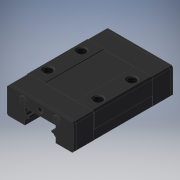
# Autodesk Inventor part: C-MLGB9
Saved by Autodesk Inventor 2019 (Build 230136000, 136)
## iProperties
Created: 2023-11-06
Part Number: C-MLGB9
Material: Generic
Catalog Web Link: www.cadenas.de
Description: C-MLGB, E-GMLGB-Economy Miniature Liner guide - Standard type - Single Block Product
Vendor: MISUMI
Document SubType Name: Modeling
Designer: psAdmin
Manufacturer: MISUMI
Mass: 3.14177 g
Surface Area: 23.9367 cm^2
Volume: 3.14177 cm^3
Density: 1 g/cm^3
Appearance: PSOLRGB-175-175-175
Category: PARTsolutions
Company: MISUMI
Title: C-MLGB9
Author: Cadenas PARTsolutions
Comments: Economy Miniature Liner guide - Standard type - Single Block Product
PSOL_IDENT_0: {$CADENAS_DATA/23d-libs/misumi/metric/06_linear_guides/c_mlgb.prj},165 {VTYP=3D},{NB=C-MLGB9},{LINA=
PSOL_IDENT_1: C-MLGB9},{NN=C-MLGB, E-GMLGB},{DATE=17.08.2023 07:57:07},{GEOMDATE=20.07.2023 00:04:58},{VERSION=},{
PSOL_IDENT_2: LINEID=20},{WBVAR=ST},{WBNUMERIC=}  {NB=C-MLGB9},{LINA=C-MLGB9},{KT=DUMMY},{PN=C-MLGB9},{TYPE=C-MLGB
PSOL_IDENT_3: },{ST=1},{NM=9},{WR=9},{H=10},{H1=2.0},{N=5.5},{W=20},{B=15},{B1=2.5},{C=10},{L1=17.5},{L2=29.60},{G
PSOL_IDENT_4: NN=Dia.1.4},{GNN3D=1.4},{M=3},{LL=3.0},{ML=M3x3},{H2=1.8},{RA1=0.45},{RA2=1.000},{RA1X=0.85},{RA2X=0
PSOL_IDENT_5: .4},{RAY=4.5},{CA1=0.2},{CA2=0.2},{BHA1=19.79},{BHA2=0.08},{BHA3=9.4},{BVA1=7.800},{BVA2=4.8},{BCA1=
PSOL_IDENT_6: 0.50},{BCA2=0.42},{BCA3=0.37},{BCA4=0.37},{BCA5=0.200},{BRA1=0.35},{BRA2=1.00},{BHB1=9.8},{BHB2=9.2}
PSOL_IDENT_7: ,{BVB1=5.0},{BVB2=4.6},{BHC1=0.80},{BRC1=0.15},{BAC1=0.72},{ML1=4.00},{ML2=0.46852},{MD1=2.459},{BHD
PSOL_IDENT_8: 1=10.0},{BHD2=0.200},{BHD3=1.75},{BHD4=0.40},{BVD1=1.8},{BRD1=2.4},{BRD2=0.15}
NB: C-MLGB9
NN: C-MLGB, E-GMLGB
NT: Economy Miniature Liner guide - Standard type - Single Block Product
NBSYN: $PN.
LINA: C-MLGB9
CATALOG: Misumi
PN: C-MLGB9
ST: No Surface Treatment
NM: 9
H: 10
H1: 2
N: 5.5
W: 20
B: 15
B1: 2.5
C: 10
L1: 17.5
L2: 29.6
GNN: Dia.1.4
ML: M3x3
H2: 1.8
SUPPLIER: MISUMI
ARTICLENO: C-MLGB9
BOMINFO: C-MLGB9
CREATOR: CADENAS GmbH
Autodesk Inventor part; units mm, degrees
sketch "_____7" plane through (0, 0, 0) normal (0, 0, 1) x (1, 0, 0)
  line L0 (-10, 9.5) -> (-10, 5.2)
  line L1 (-10, 5.2) -> (-9.92, 5.2)
  line L2 (-9.92, 5.2) -> (-9.92, 2.42)
  line L3 (-9.92, 2.42) -> (-9.5, 2)
  line L4 (-9.5, 2) -> (9.5, 2)
  line L5 (9.5, 2) -> (9.92, 2.42)
  line L6 (9.92, 2.42) -> (9.92, 5.2)
  line L7 (9.92, 5.2) -> (10, 5.2)
  line L8 (10, 5.2) -> (10, 9.5)
  line L9 (10, 9.5) -> (9.5, 10)
  line L10 (9.5, 10) -> (4.7, 10)
  line L11 (4.7, 10) -> (4.5, 9.8)
  line L12 (4.5, 9.8) -> (-4.5, 9.8)
  line L13 (-4.5, 9.8) -> (-4.7, 10)
  line L14 (-4.7, 10) -> (-9.5, 10)
  line L15 (-9.5, 10) -> (-10, 9.5)
  constraints: 32 end point
extrude "Extrusion1" add sketch "_____7" along normal mid plane 17.5
sketch "_____2" plane through (0, 0, 8.75) normal (0, 0, 1) x (1, 0, 0)
  line L0 (-9.895, 9.43) -> (-9.895, 2.37)
  line L1 (-9.895, 2.37) -> (-9.525, 2)
  line L2 (-9.525, 2) -> (9.525, 2)
  line L3 (9.525, 2) -> (9.895, 2.37)
  line L4 (9.895, 2.37) -> (9.895, 9.43)
  line L5 (9.895, 9.43) -> (9.525, 9.8)
  line L6 (9.525, 9.8) -> (-9.525, 9.8)
  line L7 (-9.525, 9.8) -> (-9.895, 9.43)
  constraints: 16 end point
extrude "Extrusion2" add sketch "_____2" along normal blind 5.25
sketch "_____8" plane through (0, 0, 14) normal (0, 0, 1) x (1, 0, 0)
  line L0 (-9.895, 9.43) -> (-9.895, 2.37)
  line L1 (-9.895, 2.37) -> (-9.525, 2)
  line L2 (-9.525, 2) -> (9.525, 2)
  line L3 (9.525, 2) -> (9.895, 2.37)
  line L4 (9.895, 2.37) -> (9.895, 9.43)
  line L5 (9.895, 9.43) -> (9.525, 9.8)
  line L6 (9.525, 9.8) -> (-9.525, 9.8)
  line L7 (-9.525, 9.8) -> (-9.895, 9.43)
  constraints: 16 end point
extrude "Extrusion3" add sketch "_____8" along normal blind 0.8 draft -0.72
sketch "_____3" plane through (0, 0, -8.75) normal (0, 0, 1) x (1, 0, 0)
  line L0 (-9.895, 9.43) -> (-9.895, 2.37)
  line L1 (-9.895, 2.37) -> (-9.525, 2)
  line L2 (-9.525, 2) -> (9.525, 2)
  line L3 (9.525, 2) -> (9.895, 2.37)
  line L4 (9.895, 2.37) -> (9.895, 9.43)
  line L5 (9.895, 9.43) -> (9.525, 9.8)
  line L6 (9.525, 9.8) -> (-9.525, 9.8)
  line L7 (-9.525, 9.8) -> (-9.895, 9.43)
  constraints: 16 end point
extrude "Extrusion4" add sketch "_____3" against normal blind 5.25
sketch "_____9" plane through (0, 0, -14) normal (0, 0, 1) x (1, 0, 0)
  line L0 (-9.895, 9.43) -> (-9.895, 2.37)
  line L1 (-9.895, 2.37) -> (-9.525, 2)
  line L2 (-9.525, 2) -> (9.525, 2)
  line L3 (9.525, 2) -> (9.895, 2.37)
  line L4 (9.895, 2.37) -> (9.895, 9.43)
  line L5 (9.895, 9.43) -> (9.525, 9.8)
  line L6 (9.525, 9.8) -> (-9.525, 9.8)
  line L7 (-9.525, 9.8) -> (-9.895, 9.43)
  constraints: 16 end point
extrude "Extrusion5" add sketch "_____9" against normal blind 0.8 draft -0.72
sketch "_____4" plane through (0, 0, 0) normal (0, 0, 1) x (1, 0, 0)
  arc A0 (-4.9, 5.5) -> (-4.9, 3.5) centre (-4.9, 4.5) ccw
  line L0 (-4.9, 3.5) -> (-4.9, 2)
  line L1 (-4.9, 2) -> (4.9, 2)
  line L2 (4.9, 2) -> (4.9, 3.5)
  arc A1 (4.9, 3.5) -> (4.9, 5.5) centre (4.9, 4.5) ccw
  line L3 (4.9, 5.5) -> (4.9, 7)
  line L4 (4.9, 7) -> (-4.9, 7)
  line L5 (-4.9, 7) -> (-4.9, 5.5)
  constraints: 12 end point, 4 point on circle, 2 centre point
extrude "Extrusion6" cut sketch "_____4" along normal mid plane 17.5
sketch "_____5" plane through (0, 0, 8.75) normal (0, 0, 1) x (1, 0, 0)
  line L0 (-4.6, 2) -> (4.6, 2)
  line L1 (4.6, 2) -> (4.6, 3.5461)
  arc A0 (3.9633, 4.15) -> (4.6, 3.5461) centre (4.9, 4.5) ccw
  line L2 (3.9633, 4.15) -> (3.65, 4.15)
  arc A1 (3.65, 4.85) -> (3.65, 4.15) centre (3.65, 4.5) ccw
  line L3 (3.65, 4.85) -> (3.9633, 4.85)
  arc A2 (4.6, 5.4539) -> (3.9633, 4.85) centre (4.9, 4.5) ccw
  line L4 (4.6, 5.4539) -> (4.6, 6.6)
  line L5 (4.6, 6.6) -> (-4.6, 6.6)
  line L6 (-4.6, 6.6) -> (-4.6, 5.4539)
  arc A3 (-3.9633, 4.85) -> (-4.6, 5.4539) centre (-4.9, 4.5) ccw
  line L7 (-3.9633, 4.85) -> (-3.65, 4.85)
  arc A4 (-3.65, 4.15) -> (-3.65, 4.85) centre (-3.65, 4.5) ccw
  line L8 (-3.65, 4.15) -> (-3.9633, 4.15)
  arc A5 (-4.6, 3.5461) -> (-3.9633, 4.15) centre (-4.9, 4.5) ccw
  line L9 (-4.6, 3.5461) -> (-4.6, 2)
  constraints: 20 end point, 12 point on circle, 6 centre point
extrude "Extrusion7" cut sketch "_____5" along normal blind 6.05
sketch "_____6" plane through (0, 0, -8.75) normal (0, 0, 1) x (1, 0, 0)
  line L0 (-4.6, 2) -> (4.6, 2)
  line L1 (4.6, 2) -> (4.6, 3.5461)
  arc A0 (3.9633, 4.15) -> (4.6, 3.5461) centre (4.9, 4.5) ccw
  line L2 (3.9633, 4.15) -> (3.65, 4.15)
  arc A1 (3.65, 4.85) -> (3.65, 4.15) centre (3.65, 4.5) ccw
  line L3 (3.65, 4.85) -> (3.9633, 4.85)
  arc A2 (4.6, 5.4539) -> (3.9633, 4.85) centre (4.9, 4.5) ccw
  line L4 (4.6, 5.4539) -> (4.6, 6.6)
  line L5 (4.6, 6.6) -> (-4.6, 6.6)
  line L6 (-4.6, 6.6) -> (-4.6, 5.4539)
  arc A3 (-3.9633, 4.85) -> (-4.6, 5.4539) centre (-4.9, 4.5) ccw
  line L7 (-3.9633, 4.85) -> (-3.65, 4.85)
  arc A4 (-3.65, 4.15) -> (-3.65, 4.85) centre (-3.65, 4.5) ccw
  line L8 (-3.65, 4.15) -> (-3.9633, 4.15)
  arc A5 (-4.6, 3.5461) -> (-3.9633, 4.15) centre (-4.9, 4.5) ccw
  line L9 (-4.6, 3.5461) -> (-4.6, 2)
  constraints: 20 end point, 12 point on circle, 6 centre point
extrude "Extrusion8" cut sketch "_____6" against normal blind 6.05
sketch "_____10" plane through (0, 0, 0) normal (1, 0, 0) x (0, 0, -1)
  line L0 (-14.8, 8.2) -> (-14, 8.2)
  line L1 (-14, 8.2) -> (-14, 7.5)
  line L2 (-14, 7.5) -> (-14.65, 7.5)
  arc A0 (-14.65, 7.5) -> (-14.8, 7.35) centre (-14.65, 7.35) ccw
  line L3 (-14.8, 7.35) -> (-14.8, 8.2)
  line L4 (-14.8, 8.2) -> (-14, 8.2)
  constraints: 10 end point, 2 point on circle, 1 centre point
revolve "Revolution1" cut sketch "_____10" angle 360 about axis through (0, 8.2, 14.8) along (0, 0, 1)
sketch "_____11" plane through (0, 0, 0) normal (1, 0, 0) x (0, 0, -1)
  line L0 (14, 8.2) -> (14.8, 8.2)
  line L1 (14.8, 8.2) -> (14.8, 7.35)
  arc A0 (14.8, 7.35) -> (14.65, 7.5) centre (14.65, 7.35) ccw
  line L2 (14.65, 7.5) -> (14, 7.5)
  line L3 (14, 7.5) -> (14, 8.2)
  line L4 (14, 8.2) -> (14.8, 8.2)
  constraints: 10 end point, 2 point on circle, 1 centre point
revolve "Revolution2" cut sketch "_____11" angle 360 about axis through (0, 8.2, -14) along (0, 0, 1)
sketch "Sketch11" plane through (4.7, 10, 8.75) normal (0, 1, 0) x (1, 0, 0)
  point P0 (2.8, 3.75)
hole "Hole1" at (7.5, 10, 5) direction (0, -1, 0) diameter 2.459 depth 4 tip angle 118 countersink diameter 3 countersink angle 90 thread size "M3x0.5" class "6H" standard "ISO Metric profile"
pattern_linear "Rectangular Pattern1" count 2 spacing 10 along (0, 0, -1) count 2 spacing 15 along (-1, 0, 0) of "Hole1"
sketch "_____73" plane through (0, 0, 8.75) normal (0, 0, 1) x (1, 0, 0)
  line L0 (-9.895, 9.43) -> (-9.895, 2.37)
  line L1 (-9.895, 2.37) -> (-9.525, 2)
  line L2 (-9.525, 2) -> (9.525, 2)
  line L3 (9.525, 2) -> (9.895, 2.37)
  line L4 (9.895, 2.37) -> (9.895, 9.43)
  line L5 (9.895, 9.43) -> (9.525, 9.8)
  line L6 (9.525, 9.8) -> (-9.525, 9.8)
  line L7 (-9.525, 9.8) -> (-9.895, 9.43)
  line L8 (-9.845, 9.4093) -> (-9.845, 2.3907)
  line L9 (-9.845, 2.3907) -> (-9.5043, 2.05)
  line L10 (-9.5043, 2.05) -> (9.5043, 2.05)
  line L11 (9.5043, 2.05) -> (9.845, 2.3907)
  line L12 (9.845, 2.3907) -> (9.845, 9.4093)
  line L13 (9.845, 9.4093) -> (9.5043, 9.75)
  line L14 (9.5043, 9.75) -> (-9.5043, 9.75)
  line L15 (-9.5043, 9.75) -> (-9.845, 9.4093)
  constraints: 32 end point
extrude "Extrusion9" cut sketch "_____73" along normal blind 0.05
sketch "_____74" plane through (0, 0, -8.75) normal (0, 0, 1) x (1, 0, 0)
  line L0 (-9.895, 9.43) -> (-9.895, 2.37)
  line L1 (-9.895, 2.37) -> (-9.525, 2)
  line L2 (-9.525, 2) -> (9.525, 2)
  line L3 (9.525, 2) -> (9.895, 2.37)
  line L4 (9.895, 2.37) -> (9.895, 9.43)
  line L5 (9.895, 9.43) -> (9.525, 9.8)
  line L6 (9.525, 9.8) -> (-9.525, 9.8)
  line L7 (-9.525, 9.8) -> (-9.895, 9.43)
  line L8 (-9.845, 9.4093) -> (-9.845, 2.3907)
  line L9 (-9.845, 2.3907) -> (-9.5043, 2.05)
  line L10 (-9.5043, 2.05) -> (9.5043, 2.05)
  line L11 (9.5043, 2.05) -> (9.845, 2.3907)
  line L12 (9.845, 2.3907) -> (9.845, 9.4093)
  line L13 (9.845, 9.4093) -> (9.5043, 9.75)
  line L14 (9.5043, 9.75) -> (-9.5043, 9.75)
  line L15 (-9.5043, 9.75) -> (-9.845, 9.4093)
  constraints: 32 end point
extrude "Extrusion10" cut sketch "_____74" against normal blind 0.05
sketch "_____18" plane through (0, 8.2, 0) normal (0, 1, 0) x (1, 0, 0)
  line L0 (5, -15) -> (5, -14.8)
  line L1 (5, -14.8) -> (6.2, -14.8)
  line L2 (6.2, -14.8) -> (6.2, -14.85)
  arc A0 (6.05, -15) -> (6.2, -14.85) centre (6.05, -14.85) ccw
  line L3 (6.05, -15) -> (5, -15)
  line L4 (5, -15) -> (5, -14.8)
  constraints: 10 end point, 2 point on circle, 1 centre point
revolve "Revolution3" add sketch "_____18" angle 360 about axis through (5, 8.2, 15) along (0, 0, 1)
pattern_linear "Rectangular Pattern2" count 2 spacing 10 along (-1, 0, 0) of "Revolution3"
sketch "_____20" plane through (0, 8.2, 0) normal (0, 1, 0) x (1, 0, 0)
  line L0 (5, 14.8) -> (5, 15)
  line L1 (5, 15) -> (6.05, 15)
  arc A0 (6.2, 14.85) -> (6.05, 15) centre (6.05, 14.85) ccw
  line L2 (6.2, 14.85) -> (6.2, 14.8)
  line L3 (6.2, 14.8) -> (5, 14.8)
  line L4 (5, 14.8) -> (5, 15)
  constraints: 10 end point, 2 point on circle, 1 centre point
revolve "Revolution4" add sketch "_____20" angle 360 about axis through (5, 8.2, -14.8) along (0, 0, 1)
pattern_linear "Rectangular Pattern3" count 2 spacing 10 along (-1, 0, 0) of "Revolution4"
sketch "_____22" plane through (5, 8.2, 15) normal (0, 0, 1) x (1, 0, 0)
  line L0 (-0.7601, -0.4773) -> (-0.4773, -0.7601)
  line L1 (-0.4773, -0.7601) -> (0, -0.2828)
  line L2 (0, -0.2828) -> (0.4773, -0.7601)
  line L3 (0.4773, -0.7601) -> (0.7601, -0.4773)
  line L4 (0.7601, -0.4773) -> (0.2828, 0)
  line L5 (0.2828, 0) -> (0.7601, 0.4773)
  line L6 (0.7601, 0.4773) -> (0.4773, 0.7601)
  line L7 (0.4773, 0.7601) -> (0, 0.2828)
  line L8 (0, 0.2828) -> (-0.4773, 0.7601)
  line L9 (-0.4773, 0.7601) -> (-0.7601, 0.4773)
  line L10 (-0.7601, 0.4773) -> (-0.2828, 0)
  line L11 (-0.2828, 0) -> (-0.7601, -0.4773)
  constraints: 24 end point
extrude "Extrusion11" cut sketch "_____22" against normal blind 0.2
pattern_linear "Rectangular Pattern4" count 2 spacing 10 along (-1, 0, 0) of "Extrusion11"
sketch "_____24" plane through (5, 8.2, -15) normal (0, 0, -1) x (1, 0, 0)
  line L0 (-0.7601, -0.4773) -> (-0.4773, -0.7601)
  line L1 (-0.4773, -0.7601) -> (0, -0.2828)
  line L2 (0, -0.2828) -> (0.4773, -0.7601)
  line L3 (0.4773, -0.7601) -> (0.7601, -0.4773)
  line L4 (0.7601, -0.4773) -> (0.2828, 0)
  line L5 (0.2828, 0) -> (0.7601, 0.4773)
  line L6 (0.7601, 0.4773) -> (0.4773, 0.7601)
  line L7 (0.4773, 0.7601) -> (0, 0.2828)
  line L8 (0, 0.2828) -> (-0.4773, 0.7601)
  line L9 (-0.4773, 0.7601) -> (-0.7601, 0.4773)
  line L10 (-0.7601, 0.4773) -> (-0.2828, 0)
  line L11 (-0.2828, 0) -> (-0.7601, -0.4773)
  constraints: 24 end point
extrude "Extrusion12" cut sketch "_____24" against normal blind 0.2
pattern_linear "Rectangular Pattern5" count 2 spacing 10 along (-1, 0, 0) of "Extrusion12"
ref_plane "to_rail_XY" through (0, 0, 0) normal (0, 0, -1) x (1, 0, 0)
ref_plane "to_rail_YZ" through (0, 0, 0) normal (1, 0, 0) x (0, -1, 0)
ref_plane "to_rail_ZX" through (0, 0, 0) normal (0, -1, 0) x (0, 0, -1)
body "Solid1"
